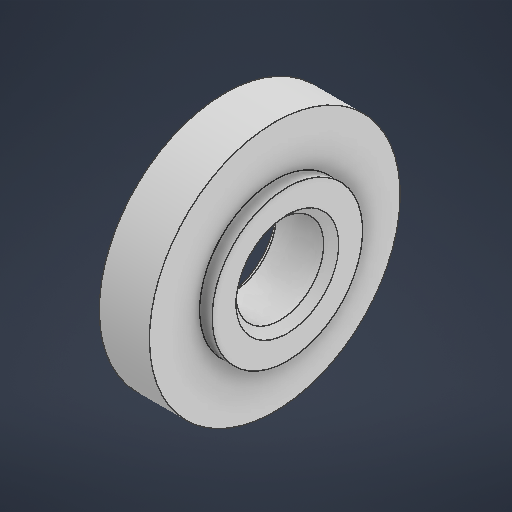
# Autodesk Inventor part: Стопорная шайба
Saved by Autodesk Inventor 2025 (Build 290162010, 162A)
## iProperties
Created: 2024-12-06
Part Number: Стопорная шайба
Material: Типовые
Document SubType Name: Modeling
Designer: Edward_Higgins
Density: 1 g/cm^3
Appearance: По умолчанию
Author: Edward_Higgins
Autodesk Inventor part; units mm, degrees
ref_plane "YZ Plane" through (0, 0, 0) normal (1, 0, 0) x (0, 1, 0)
ref_plane "XZ Plane" through (0, 0, 0) normal (0, 1, 0) x (-1, 0, 0)
ref_plane "XY Plane" through (0, 0, 0) normal (0, 0, 1) x (1, 0, 0)
sketch "Эскиз1" plane through (0, 0, 0) normal (0, 0, 1) x (1, 0, 0)
  line L0 (0, 1.75) -> (0, 3)
  line L1 (0, 3) -> (-0.5, 3)
  line L2 (-0.5, 3) -> (-0.5, 5)
  line L3 (-0.5, 5) -> (-2.5, 5)
  line L4 (-2.5, 5) -> (-2.5, 1.75)
  line L5 (-2.5, 1.75) -> (0, 1.75)
  line L6 (0, 0) -> (-4.5246, 0) construction
  dimension "d0" = 6
  dimension "d1" = 10
  dimension "d2" = 3.5
  dimension "d3" = 0.5
  dimension "d12" = 2
  constraints: 14 end point, 3 perpendicular, 2 vertical, 1 horizontal, 1 parallel, 1 vertical alignment
  measures "d0" diameter of L1 L6
  measures "d1" diameter of L3 L6
  measures "d2" diameter of L5 L6
  measures "d3" distance between parallel lines of L0 L2
  measures "d12" distance between parallel lines of L2 L4
revolve "Вращение1" add sketch "Эскиз1" angle 360 about axis through (0, 0, 0) along (-1, 0, 0)
chamfer "Фаска1" distance 0.3 angle 45 2 edges at (-2.5, -1.75, 0) (0, -1.75, 0)
